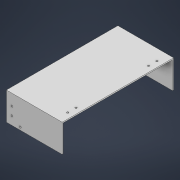
# Autodesk Inventor part: Ebene3_mitte_vorne
Saved by Autodesk Inventor 2021 (Build 250183000, 183)
## iProperties
Created: 2021-02-07
Part Number: Ebene3_mitte_vorne
Material: Generisch
Document SubType Name: Modeling
Designer: laure
Density: 1 g/cm^3
Appearance: Vorgabe
Author: laure
## iProperties of the stored document _3D-Druck.ipt
Created: 2021-03-02
Part Number: _3D-Druck
Material: Generisch
Document SubType Name: Modeling
Designer: Ctroi
Density: 1 g/cm^3
Appearance: Vorgabe
Author: Ctroi
Autodesk Inventor part; units mm, degrees
ref_plane "YZ Plane" through (0, 0, 0) normal (1, 0, 0) x (0, 1, 0)
ref_plane "XZ Plane" through (0, 0, 0) normal (0, 1, 0) x (-1, 0, 0)
ref_plane "XY Plane" through (0, 0, 0) normal (0, 0, 1) x (1, 0, 0)
sketch "Skizze1" plane through (0, 0, 0) normal (0, 1, 0) x (-1, 0, 0)
  line L0 (50, -100) -> (-50, -100)
  line L1 (-50, -100) -> (-50, 100)
  line L2 (-50, 100) -> (50, 100)
  line L3 (50, 100) -> (50, -100)
  line L4 (0, -140) -> (0, 140) projected
  line L5 (70, 0) -> (-70, 0) projected
  point P0 (0, 0)
  dimension "d0" = 100
  dimension "d1" = 200
  constraints: 8 end point, 2 parallel, 1 horizontal, 1 perpendicular, 2 other
  measures "d0" distance between parallel lines of L1 L3
  measures "d1" distance between parallel lines of L2 L0
extrude "Extrusion1" add sketch "Skizze1" along normal mid plane 2
sketch "Skizze3" plane through (0, -1, 0) normal (0, -1, 0) x (1, 0, 0)
  line L0 (50, -100) -> (-50, -100) projected
  line L1 (-50, -100) -> (-50, 100) projected
  line L2 (50, -100) -> (-50, -100)
  line L3 (-50, -100) -> (-50, -98)
  line L4 (-50, -98) -> (50, -98)
  line L5 (50, -98) -> (50, -100)
  line L6 (50, 100) -> (50, -100) projected
  line L7 (50, 100) -> (-50, 100)
  line L8 (-50, 100) -> (-50, 98)
  line L9 (-50, 98) -> (50, 98)
  line L10 (50, 98) -> (50, 100)
  point P0 (0, 0)
  dimension "d8" = 2
  dimension "d9" = 2
  constraints: 16 end point, 4 parallel, 2 horizontal, 2 perpendicular, 2 point on line
  measures "d8" distance of L2.end L3.end
  measures "d9" distance of L8.end L7.end
extrude "Extrusion3" add sketch "Skizze3" along normal blind 48 contours L0 L1 L4 L5 | L9 L1 L7 L6
sketch "Skizze4" plane through (-50, 1, 100) normal (0, 0, 1) x (1, 0, 0)
  circle A0 centre (10, -20) radius 1.6
  circle A1 centre (10, -35) radius 1.6
  line L0 (100, -50) -> (0, -50) projected
  line L1 (0, -50) -> (0, 0) projected
  point P0 (50, -1)
  dimension "d12" = 3.2
  dimension "d13" = 3.2
  dimension "d14" = 15
  dimension "d15" = 15
  dimension "d16" = 10
  dimension "d17" = 10
  constraints: 2 centre point
  measures "d12" diameter of A0
  measures "d13" diameter of A1
  measures "d14" distance from line of A1.centre L0
  measures "d15" distance of A0.centre A1.centre
  measures "d16" distance from line of L1 A0.centre
  measures "d17" distance from line of L1 A1.centre
extrude "Extrusion4" cut sketch "Skizze4" against normal up to surface (2 mm away)
sketch "Skizze5" plane through (50, 1, -100) normal (0, 0, -1) x (-1, 0, 0)
  circle A0 centre (90, -20) radius 1.6
  circle A1 centre (90, -35) radius 1.6
  line L0 (100, -50) -> (100, 0) projected
  line L1 (100, -50) -> (0, -50) projected
  point P0 (50, -1)
  dimension "d20" = 3.2
  dimension "d21" = 3.2
  dimension "d22" = 10
  dimension "d23" = 10
  dimension "d24" = 15
  dimension "d25" = 15
  constraints: 2 centre point
  measures "d20" diameter of A0
  measures "d21" diameter of A1
  measures "d22" distance from line of L0 A1.centre
  measures "d23" distance from line of L0 A0.centre
  measures "d24" distance from line of L1 A1.centre
  measures "d25" distance of A1.centre A0.centre
extrude "Extrusion5" cut sketch "Skizze5" against normal up to surface (2 mm away)
sketch "Skizze6" plane through (0, 1, 0) normal (0, 1, 0) x (1, 0, 0)
  line L0 (50, -100) -> (50, 100) projected
  circle A0 centre (40, -65) radius 1.6
  circle A1 centre (40, -80) radius 1.6
  circle A2 centre (40, 80) radius 1.6
  circle A3 centre (40, 65) radius 1.6
  line L1 (-50, -100) -> (50, -100) projected
  line L2 (50, 100) -> (-50, 100) projected
  point P0 (0, 0)
  dimension "d31" = 3.2
  dimension "d32" = 3.2
  dimension "d33" = 3.2
  dimension "d34" = 3.2
  dimension "d35" = 10
  dimension "d36" = 10
  dimension "d37" = 15
  dimension "d38" = 10
  dimension "d39" = 10
  dimension "d40" = 15
  dimension "d41" = 20
  dimension "d42" = 20
  constraints: 4 centre point
  measures "d31" diameter of A0
  measures "d32" diameter of A1
  measures "d33" diameter of A2
  measures "d34" diameter of A3
  measures "d35" distance from line of A0.centre L0
  measures "d36" distance from line of A1.centre L0
  measures "d37" distance of A1.centre A0.centre
  measures "d38" distance from line of L0 A2.centre
  measures "d39" distance from line of L0 A3.centre
  measures "d40" distance of A2.centre A3.centre
  measures "d41" distance from line of A1.centre L1
  measures "d42" distance from line of L2 A2.centre
extrude "Extrusion6" cut sketch "Skizze6" against normal up to surface (2 mm away)
sketch "Skizze7" plane through (-50, 1, 100) normal (0, 0, 1) x (1, 0, 0)
  circle A0 centre (25, -45) radius 1.6
  line L0 (0, -50) -> (0, 0) projected
  line L1 (100, -50) -> (0, -50) projected
  point P0 (50, -1)
  dimension "d45" = 3.2
  dimension "d46" = 25
  dimension "d47" = 5
  constraints: 1 centre point
  measures "d45" diameter of A0
  measures "d46" distance from line of A0.centre L0
  measures "d47" distance from line of A0.centre L1
extrude "Extrusion7" cut sketch "Skizze7" against normal up to surface (2 mm away)
sketch "Skizze8" plane through (50, 1, -100) normal (0, 0, -1) x (-1, 0, 0)
  circle A0 centre (75, -45) radius 1.6
  line L0 (100, -50) -> (100, 0) projected
  line L1 (100, -50) -> (0, -50) projected
  point P0 (50, -1)
  dimension "d50" = 3.2
  dimension "d51" = 25
  dimension "d52" = 5
  constraints: 1 centre point
  measures "d50" diameter of A0
  measures "d51" distance from line of A0.centre L0
  measures "d52" distance from line of L1 A0.centre
extrude "Extrusion8" cut sketch "Skizze8" against normal up to surface (2 mm away)
